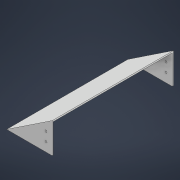
# Autodesk Inventor part: Ebene3_vorne
Saved by Autodesk Inventor 2021 (Build 250183000, 183)
## iProperties
Created: 2021-02-07
Part Number: Ebene3_vorne
Material: Generisch
Document SubType Name: Modeling
Designer: laure
Density: 1 g/cm^3
Appearance: Vorgabe
Author: laure
## iProperties of the stored document _3D-Druck.ipt
Created: 2021-03-02
Part Number: _3D-Druck
Material: Generisch
Document SubType Name: Modeling
Designer: Ctroi
Density: 1 g/cm^3
Appearance: Vorgabe
Author: Ctroi
Autodesk Inventor part; units mm, degrees
ref_plane "YZ Plane" through (0, 0, 0) normal (1, 0, 0) x (0, 1, 0)
ref_plane "XZ Plane" through (0, 0, 0) normal (0, 1, 0) x (-1, 0, 0)
ref_plane "XY Plane" through (0, 0, 0) normal (0, 0, 1) x (1, 0, 0)
sketch "Skizze1" plane through (0, 0, 0) normal (0, 0, 1) x (1, 0, 0)
  line L0 (-50, -25) -> (25, 25)
  line L1 (25, 25) -> (25, -25)
  line L2 (25, -25) -> (-50, -25)
  line L3 (0, 35) -> (0, -35) projected
  line L4 (-65, 0) -> (40, 0) projected
  line L5 (23, 21.263) -> (-43.3944, -23)
  line L6 (-43.3944, -23) -> (23, -23)
  line L7 (23, -23) -> (23, 21.263)
  line L8 (23, -23) -> (25, -23)
  line L9 (25, 22.5963) -> (23, 21.263)
  line L10 (-43.3944, -23) -> (-46.3944, -25)
  point P0 (0, 0)
  dimension "d0" = 50
  dimension "d1" = 75
  dimension "d2" = 25
  dimension "d3" = 25
  dimension "d4" = 2
  constraints: 18 end point, 4 point on line, 3 perpendicular, 1 collinear, 1 vertical, 2 other
  measures "d0" distance of L0.end L1.end
  measures "d1" distance from line of L0.start L1
  measures "d2" distance between parallel lines of L4 L2
  measures "d3" distance between parallel lines of L3 L1
  measures "d4" distance between parallel lines of L0 L5
extrude "Extrusion2" add sketch "Skizze1" along normal mid plane 200 contours L0 L4 L5 L10 L2 | L0 L3 L5 L4 | L0 L1 L9 L5 L3
sketch "Skizze2" plane through (0, 0, 100) normal (0, 0, 1) x (1, 0, 0)
  line L0 (-46.3944, -25) -> (25, 22.5963) projected
  line L1 (-46.3944, -25) -> (25, -25)
  line L2 (25, -25) -> (25, 22.5963)
  line L3 (25, 22.5963) -> (-46.3944, -25)
  line L4 (25, 25) -> (-50, -25) projected
  point P0 (0, 0)
  constraints: 6 end point, 1 horizontal, 1 parallel, 1 perpendicular
extrude "Extrusion3" add sketch "Skizze2" against normal blind 2
sketch "Skizze3" plane through (0, 0, -100) normal (0, 0, -1) x (-1, 0, 0)
  line L0 (-25, 22.5963) -> (46.3944, -25) projected
  line L1 (46.3944, -25) -> (50, -25) projected
  line L2 (-25, 22.5963) -> (46.3944, -25)
  line L3 (46.3944, -25) -> (-25, -25)
  line L4 (-25, -25) -> (-25, 22.5963)
  line L5 (-25, -25) -> (-25, 25) projected
  point P0 (0, 0)
  constraints: 6 end point, 2 collinear
extrude "Extrusion4" add sketch "Skizze3" against normal blind 2
sketch "Skizze4" plane through (0, 0, 100) normal (0, 0, 1) x (1, 0, 0)
  circle A0 centre (15, 5) radius 1.6
  circle A1 centre (15, -10) radius 1.6
  line L0 (-50, -25) -> (25, -25) projected
  line L1 (25, -25) -> (25, 25) projected
  point P0 (0, 0)
  dimension "d13" = 3.2
  dimension "d14" = 3.2
  dimension "d15" = 15
  dimension "d16" = 15
  dimension "d17" = 10
  dimension "d18" = 10
  constraints: 2 centre point
  measures "d13" diameter of A0
  measures "d14" diameter of A1
  measures "d15" distance of A0.centre A1.centre
  measures "d16" distance from line of L0 A1.centre
  measures "d17" distance from line of L1 A1.centre
  measures "d18" distance from line of L1 A0.centre
extrude "Extrusion5" cut sketch "Skizze4" against normal up to surface (2 mm away)
sketch "Skizze5" plane through (0, 0, -100) normal (0, 0, -1) x (-1, 0, 0)
  circle A0 centre (-15, 5) radius 1.6
  circle A1 centre (-15, -10) radius 1.6
  line L0 (-25, 25) -> (-25, -25) projected
  line L1 (-25, -25) -> (50, -25) projected
  point P0 (0, 0)
  dimension "d21" = 3.2
  dimension "d22" = 3.2
  dimension "d23" = 10
  dimension "d24" = 10
  dimension "d25" = 15
  dimension "d26" = 15
  constraints: 2 centre point
  measures "d21" diameter of A0
  measures "d22" diameter of A1
  measures "d23" distance from line of A0.centre L0
  measures "d24" distance from line of A1.centre L0
  measures "d25" distance from line of A1.centre L1
  measures "d26" distance of A0.centre A1.centre
extrude "Extrusion6" cut sketch "Skizze5" against normal up to surface (2 mm away)
